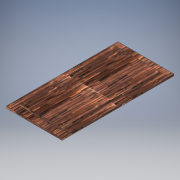
# Autodesk Inventor part: tabletop
Saved by Autodesk Inventor 2019 (Build 230136000, 136)
## iProperties
Created: 2019-08-11
Part Number: tabletop
Material: Walnut
Document SubType Name: Modeling
Designer: Alex
Density: 1 g/cm^3
Appearance: Generic
Author: Alex
Autodesk Inventor part; units mm, degrees
ref_plane "YZ Plane" through (0, 0, 0) normal (1, 0, 0) x (0, 1, 0)
ref_plane "XZ Plane" through (0, 0, 0) normal (0, 1, 0) x (-1, 0, 0)
ref_plane "XY Plane" through (0, 0, 0) normal (0, 0, 1) x (1, 0, 0)
sketch "Sketch1" plane through (0, 0, 0) normal (0, 1, 0) x (-1, 0, 0)
  line L0 (0, 0) -> (-800, 0)
  line L1 (-800, 0) -> (-800, -1600)
  line L2 (-800, -1600) -> (0, -1600)
  line L3 (0, -1600) -> (0, 0)
  dimension "d0" = 800
  dimension "d1" = 1600
  constraints: 8 end point, 2 parallel, 1 horizontal, 1 perpendicular
  measures "d0" distance of L2.end L1.end
  measures "d1" distance of L1.end L0.end
extrude "Extrusion1" add sketch "Sketch1" along normal blind 26
sketch "Sketch2" plane through (0, 26, 0) normal (0, 1, 0) x (1, 0, 0)
  line L0 (100, 100) -> (700, 100)
  line L1 (700, 100) -> (700, 1500)
  line L2 (700, 1500) -> (100, 1500)
  line L3 (100, 1500) -> (100, 100)
  line L4 (0, 1600) -> (0, 0) projected
  line L5 (800, 0) -> (800, 1600) projected
  line L6 (0, 0) -> (800, 0) projected
  line L7 (800, 1600) -> (0, 1600) projected
  dimension "d4" = 100
  dimension "d5" = 100
  dimension "d6" = 100
  dimension "d7" = 100
  constraints: 8 end point, 2 parallel, 1 horizontal, 1 perpendicular
  measures "d4" distance between parallel lines of L3 L4
  measures "d5" distance between parallel lines of L5 L1
  measures "d6" distance between parallel lines of L6 L0
  measures "d7" distance between parallel lines of L7 L2
extrude "Extrusion2" add sketch "Sketch2" along normal blind 26 contours L3 L2 L1 L0
body "Solid1"
